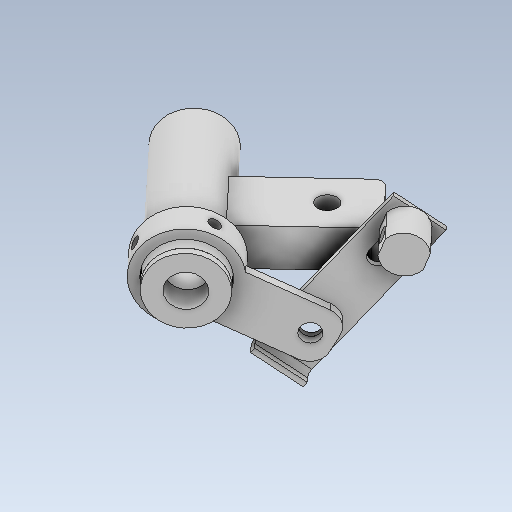
# Autodesk Inventor part: axle_eq
Saved by Autodesk Inventor 2021 (Build 250183000, 183)
## iProperties
Created: 2023-11-16
Part Number: axle_eq
Material: Generic
Document SubType Name: Modeling
Designer: vtoth
Density: 1 g/cm^3
Appearance: Default
Author: vtoth
Autodesk Inventor part; units mm, degrees
ref_plane "YZ Plane" through (0, 0, 0) normal (1, 0, 0) x (0, 1, 0)
ref_plane "XZ Plane" through (0, 0, 0) normal (0, 1, 0) x (-1, 0, 0)
ref_plane "XY Plane" through (0, 0, 0) normal (0, 0, 1) x (1, 0, 0)
derived "polus.ipt"
derived "skeleton_1.ipt"
sketch "Sketch1" plane through (0, 0, 0) normal (0, 1, 0) x (-1, 0, 0)
  line L0 (0, 0) -> (0, 550)
  circle A0 centre (0, 550) radius 6
  line L1 (0, 550) -> (43.8812, 590.9199)
  line L2 (-15.7936, 654.9134) -> (83.0961, 548.8671)
  line L3 (111.4949, 533.0759) -> (80.291, 566.538)
  line L4 (96.8679, 519.4359) -> (65.6639, 552.898)
  line L5 (0, 0) -> (-350, 0)
  line L6 (11.0017, 632.044) -> (5.1509, 626.588)
  point P0 (0, 440)
sketch "Sketch2" plane through (15.7936, 0, 654.9134) normal (-0.6819984, 0, -0.7313537) x (0, -1, 0)
  line L0 (0, -60) -> (0, 0) construction
  line L1 (-69.5467, -18.635) -> (77.2741, 20.7055)
  circle A0 centre (0, 0) radius 10
  line L2 (20.1846, -4.9443) -> (20.2151, -4.9361)
  line L3 (-20.2054, 4.9388) -> (-20.1742, 4.9471)
  line L4 (69.2185, 23.7234) -> (71.8067, 14.0642)
  point P0 (0, 0)
  point P1 (0, 0)
  point P2 (0, 0)
  point P3 (0, 10)
  point P4 (0, 10)
  point P5 (0, 10)
  point P6 (-55.0578, -14.7527)
  point P7 (43.4667, 11.6469)
ref_plane "Work Plane1" through (15.7936, 0, 654.9134) normal (-0.6819984, 0, -0.7313537) x (0, -1, 0)
ref_plane "Work Plane2" through (0.6506, -77.2741, 669.0345) normal (-0.1892883, -0.9659258, 0.1765142) x (0.9813346, -0.1923079, 0)
sketch "Sketch4_1" plane through (15.7936, 0, 654.9134) normal (-0.1892883, 0.9659258, 0.1765142) x (-0.6819984, 0, -0.7313537)
  line L0 (0, 0) -> (145, 0) construction
  line L1 (45, 0) -> (45, -99)
  line L2 (45, -99) -> (39, -99)
sketch "Sketch6" plane through (59.1326, 25.6231, 561.1733) normal (0.25013, 0.9396965, -0.23325) x (-0.6819984, 0, -0.7313537)
  line L0 (6, 0) -> (0, 0) construction
  line L1 (0, 0) -> (0, 86.0639)
  line L2 (0, 86.0639) -> (-39, 86.0639)
  point P0 (-5, 86.0639)
  point P1 (4, 0)
  point P2 (-4, 0)
  point P3 (5, 86.0639)
ref_plane "Work Plane3" through (15.7936, 0, 654.9134) normal (0, 1, 0) x (-0.6819984, 0, -0.7313537)
sketch "Sketch4" plane through (15.7936, 0, 654.9134) normal (0, 1, 0) x (-0.6819984, 0, -0.7313537)
  line L0 (0, 0) -> (145, 0) projected
  line L1 (175.9169, -10) -> (130.1632, -10) construction
  line L2 (175.9169, 10) -> (130.1632, 10) construction
  line L3 (87.5, -60) -> (87.5, 0) construction
  circle A0 centre (87.5, -60) radius 6 projected
  line L4 (35, -10) -> (35, -20)
  line L5 (35, -20) -> (145, -20)
  line L6 (145, -20) -> (145, -10)
  line L7 (145, -10) -> (130, -10)
  line L8 (130, -10) -> (130, -15)
  line L9 (130, -15) -> (50, -15)
  line L10 (50, -15) -> (50, -10)
  line L11 (50, -10) -> (35, -10)
  line L12 (106, -20) -> (106, -80)
  arc A1 (101, -85) -> (106, -80) centre (101, -80) ccw
  line L13 (101, -85) -> (74, -85)
  arc A2 (69, -80) -> (74, -85) centre (74, -80) ccw
  line L14 (69, -80) -> (69, -20)
  line L15 (69, -20) -> (69, -15)
  line L16 (106, -20) -> (106, -15)
  line L17 (50, -15) -> (39, -15)
  line L18 (39, -15) -> (39, -20)
  line L19 (35, 4) -> (35, -4) construction
  point P0 (489.7445, -435.0991)
  dimension "d3" = 15
  dimension "d4" = 15
  dimension "d6" = 30
  dimension "d7" = 40
  dimension "d8" = 37
  dimension "d9" = 25
  dimension "d10" = 5
  dimension "d15" = 4
  constraints: 30 end point, 12 perpendicular, 7 point on line, 4 point on circle, 4 tangent, 3 collinear, 2 centre point, 2 symmetric about line, 1 parallel
  measures "d3" distance between parallel lines of L4 L10
  measures "d4" distance between parallel lines of L6 L8
  measures "d6" diameter of L9 L0
  measures "d7" diameter of L5 L0
  measures "d8" distance between parallel lines of L14 L12
  measures "d9" distance from line of L3.start L13
  measures "d10" radius of A1
  measures "d15" distance between parallel lines of L4 L18
extrude "Extrusion2" add sketch "Sketch4" along normal mid plane 23 contours L15 L9 L16 L5 | L5 L12 A1 L13 A2 L14
revolve "Revolution3" [suppressed]
revolve "Revolution1" add sketch "Sketch4" angle 360 about axis through (15.7936, 0, 654.9134) along (-0.6819984, 0, -0.7313537) contours L18 L17 L9 L15 L5 | L15 L9 L16 L5 | L16 L9 L8 L7 L6 L5
revolve "Revolution2" add sketch "Sketch4" angle 360 about axis through (15.7936, 0, 654.9134) along (-0.6819984, 0, -0.7313537) separate body contours L11 L10 L17 L18 L5 L4
ref_plane "Work Plane4" through (-14.8963, 0, 622.0024) normal (-0.6819984, 0, -0.7313537) x (0, -1, 0)
sketch "Sketch7" plane through (-14.8963, 0, 622.0024) normal (-0.6819984, 0, -0.7313537) x (0, -1, 0)
  circle A0 centre (0, 0) radius 20 construction
  line L0 (0, 0) -> (-25.6231, -95.6267) construction
  circle A1 centre (0, 0) radius 20.5
  circle A2 centre (0, 0) radius 26
  line L1 (0, 0) -> (28.212, -54.0841) construction
  line L2 (28.212, -54.0841) -> (-25.6231, -95.6267) construction
  line L3 (23.1212, -11.8917) -> (42.4363, -48.9199)
  arc A3 (38.195, -62.4111) -> (42.4363, -48.9199) centre (33.5701, -53.5448) ccw
  line L4 (38.195, -62.4111) -> (29.3287, -67.036)
  arc A4 (15.8376, -62.7947) -> (29.3287, -67.036) centre (24.7038, -58.1698) ccw
  line L5 (15.8376, -62.7947) -> (-3.4775, -25.7664)
  circle A5 centre (28.212, -54.0841) radius 5.5
  point P0 (0, -435.0991)
  dimension "d20" = 68
  dimension "d21" = 61
  dimension "d22" = 0.5
  dimension "d23" = 52
  dimension "d24" = 30
  dimension "d25" = 47
  dimension "d26" = 10
  dimension "d27" = 11
  constraints: 10 end point, 6 point on circle, 5 centre point, 4 tangent, 3 coincident, 3 symmetric about line, 1 perpendicular
  measures "d20" distance of L1.end L0.end
  measures "d21" distance of A0.centre L1.end
  measures "d22" radial gap between concentric circles of A1 A0
  measures "d23" diameter of A2
  measures "d24" distance between parallel lines of L3 L5
  measures "d25" distance edge to line of A2 L4
  measures "d26" radius of A4
  measures "d27" diameter of A5
extrude "Extrusion3" add sketch "Sketch7" along normal blind 17 separate body contours A2
extrude "Extrusion4" add sketch "Sketch7" along normal blind 5 contours A2 L3 A3 L4 A4 L5 bodies 3
ref_plane "Work Plane5" through (-31.7556, 12.0248, 637.724) normal (0.6484357, -0.4624912, -0.604676) x (0.5806751, 0.8141354, 0)
sketch "Sketch8" plane through (-31.7556, 12.0248, 637.724) normal (0.6484357, -0.4624912, -0.604676) x (0.5806751, 0.8141354, 0)
  line L0 (-23.8743, 10.2965) -> (23.8743, -10.2965) construction
  line L1 (-30.6066, -5.3136) -> (17.142, -25.9066) construction
  line L2 (0, 0) -> (-6.7323, -15.6101) construction
  point P0 (8.6499, -488.074)
  point P1 (0, 0)
  point P2 (-3.3662, -7.8051)
  constraints: 2 end point, 2 midpoint
hole "Hole1" at (-37.5526, 12.0248, 631.5075) direction (0.6484357, -0.4624912, -0.604676) diameter 6.647 end up to face face through (-14.8963, 0, 622.0024) facing (-0.6819984, 0, -0.7313537) round with radius 20.5 far side no bodies 3 thread size "M8x1.25" class "6H" standard "ISO Metric profile"
pattern_circular "Circular Pattern1" count 2 over 270 about axis through (-14.8963, 0, 622.0024) along (-0.6819984, 0, -0.7313537) of "Hole1" bodies 3
pattern_circular "Circular Pattern2" count 2 over 90 about axis through (-14.8963, 0, 622.0024) along (-0.6819984, 0, -0.7313537) of "Hole1" bodies 3
ref_plane "Work Plane6" through (24.6583, -28.212, 585.1172) normal (0.5790068, -0.6109206, -0.5399326) x (0.446799, 0.7916919, -0.4166468)
sketch "Sketch9" plane through (24.6583, -28.212, 585.1172) normal (0.5790068, -0.6109206, -0.5399326) x (0.446799, 0.7916919, -0.4166468)
  line L0 (0, 0) -> (68, 0) construction
  line L1 (7.0285, -5) -> (-2.8163, -5) projected
  line L2 (-18, -5) -> (78, -5)
  line L3 (78, -5) -> (78, -8)
  line L4 (78, -8) -> (-18, -8)
  arc A0 (-24, -2) -> (-18, -8) centre (-18, -2) ccw
  line L5 (-24, -2) -> (-24, 1.5)
  line L6 (-24, 1.5) -> (-21, 1.5)
  line L7 (-21, 1.5) -> (-21, -2)
  arc A1 (-21, -2) -> (-18, -5) centre (-18, -2) ccw
  point P0 (255.1051, -444.7445)
  point P1 (7.0285, -5)
  point P2 (-2.8163, -5)
  dimension "d46" = 3
  dimension "d47" = 3
  dimension "d49" = 9.5
  dimension "d50" = 21
  dimension "d51" = 102
  constraints: 12 end point, 5 perpendicular, 4 point on circle, 4 tangent, 2 centre point, 1 collinear, 1 concentric
  measures "d46" distance between parallel lines of L2 L4
  measures "d47" radius of A1
  measures "d49" distance between parallel lines of L4 L6
  measures "d50" distance from line of L0.start L7
  measures "d51" distance between parallel lines of L5 L3
extrude "Extrusion5" add sketch "Sketch9" along normal mid plane 29 separate body
sketch "Sketch10" plane through (21.6015, -51.3208, 581.131) normal (0.6819984, 0, 0.7313537) x (0.446799, 0.7916919, -0.4166468)
  circle A0 centre (18, 14.5) radius 5.5 projected
  line L0 (941.2546, 14.5) -> (-312.0443, 14.5) construction
  line L1 (86, 14.5) -> (66, 14.5) construction
  line L2 (86, 19.5) -> (66, 19.5)
  line L3 (66, 9.5) -> (86, 9.5)
  arc A1 (86, 9.5) -> (86, 19.5) centre (86, 14.5) ccw
  arc A2 (66, 19.5) -> (66, 9.5) centre (66, 14.5) ccw
  point P0 (273.1051, -269.9112)
  point P1 (76, 14.5)
  dimension "d54" = 10
  dimension "d55" = 30
  constraints: 8 end point, 4 point on circle, 4 tangent, 2 centre point, 1 midpoint, 1 parallel, 1 point on line
  measures "d54" diameter of A2
extrude "Extrusion6" cut sketch "Sketch10" against normal through all bodies 4
sketch "Sketch11" plane through (24.6583, -28.212, 585.1172) normal (0.5790068, -0.6109206, -0.5399326) x (0.446799, 0.7916919, -0.4166468)
  line L0 (78, -5) -> (-18, -5) construction
  line L1 (-18, -8) -> (78, -8) construction
  line L2 (0, 0) -> (68, 0) construction
  line L3 (68, 10.1333) -> (68, -18.0749) construction
  line L4 (68, -14) -> (73, -14)
  line L5 (73, -14) -> (73, -5)
  line L6 (-18, -5) -> (78, -5) construction
  line L7 (73, -5) -> (79.5, -5)
  line L8 (79.5, -5) -> (79.5, 15.5)
  line L9 (79.5, 15.5) -> (68, 15.5)
  line L10 (68, 15.5) -> (68, -14)
  point P0 (255.1051, -444.7445)
  point P1 (79.5, 6.5)
  dimension "d58" = 10
  dimension "d59" = 23
  dimension "d60" = 6
  dimension "d61" = 20.5
  dimension "d65" = 9
  constraints: 14 end point, 6 point on line, 5 perpendicular, 1 vertical
  measures "d58" diameter of L5 L3
  measures "d59" diameter of L8 L3
  measures "d60" distance between parallel lines of L1 L4
  measures "d61" distance between parallel lines of L9 L7
  measures "d65" distance from line of point (79.5, 6.5) L9
revolve "Revolution4" add sketch "Sketch11" angle 360 about axis through (61.9515, 25.6231, 564.1963) along (-0.6819984, 0, -0.7313537) separate body
thread "Thread1" size "M10x1.5" class "6g" standard "ISO Metric profile" full length
ref_plane "Work Plane8" through (59.1326, 25.6231, 561.1733) normal (0.25013, 0.9396965, -0.23325) x (-0.6872505, 0.3420096, 0.6408715)
sketch "Sketch13" plane through (59.1326, 25.6231, 561.1733) normal (0.25013, 0.9396965, -0.23325) x (-0.6872505, 0.3420096, 0.6408715)
  line L0 (0, 0) -> (86.0639, 0) construction
  line L1 (-11.5, 9.5) -> (-11.5, -11) projected
  line L2 (11.5, 9.5) -> (11.5, -11) projected
  line L3 (11.5, 9.5) -> (10.5, 9.5)
  line L4 (10.5, 9.5) -> (10.5, -11)
  line L5 (41.7218, -8) -> (14.0879, -8) projected
  line L6 (-11.5, -11) -> (11.5, -11) projected
  line L7 (10.5, -11) -> (11.5, -11)
  line L8 (-11.5, 9.5) -> (-10.5, 9.5)
  line L9 (-10.5, 9.5) -> (-10.5, -11)
  line L10 (-10.5, -11) -> (-11.5, -11)
  point P0 (-327.7644, -450.7445)
  point P1 (-11.5, 0)
  point P2 (10.5, -11)
  point P3 (-10.5, -11)
  dimension "d73" = 1
  dimension "d74" = 1
  constraints: 12 end point, 6 perpendicular, 2 point on line
  measures "d73" distance between parallel lines of L4 L2
  measures "d74" distance between parallel lines of L1 L9
ref_plane "Work Plane7" through (67.036, 21.69, 553.8033) normal (0.6872505, -0.3420096, -0.6408715) x (0.445529, 0.8952675, 0)
sketch "Sketch12" plane through (67.036, 21.69, 553.8033) normal (0.6872505, -0.3420096, -0.6408715) x (0.445529, 0.8952675, 0)
  point P0 (-49.2848, -457.395)
  point P1 (0, 0)
hole "Hole2" at (67.036, 21.69, 553.8033) direction (-0.6872505, 0.3420096, 0.6408715) diameter 8 end through all bodies 5
extrude "Extrusion7" cut sketch "Sketch13" against normal through all both and the other way through all bodies 2 5
equation "\"d17\" = tav"
equation "\"d47\" = d46"
equation "\"d74\" = d73"
equation "\"tav\" = 23"
